Autodesk Inventor part; units mm, degrees
(part 4 of 4)
  line L785 (-17.051083, 24.790146) -> (-16.754475, 24.905018)
  line L786 (-16.754475, 24.905018) -> (-16.713136, 24.929783)
  line L787 (-16.713136, 24.929783) -> (-16.476535, 25.079515)
  line L788 (-16.476535, 25.079515) -> (-16.131349, 24.532971)
  line L789 (-16.131349, 24.532971) -> (-18.059781, 23.317391)
  line L790 (-18.059781, 23.317391) -> (-18.405157, 23.864126)
  line L791 (-18.405157, 23.864126) -> (-18.185892, 24.001666)
  line L792 (-18.185892, 24.001666) -> (-18.145696, 24.027575)
  line L793 (-18.145696, 24.027575) -> (-17.914239, 24.245697)
  line L794 (-17.914239, 24.245697) -> (-17.908905, 24.263032)
  line L795 (-17.908905, 24.263032) -> (-17.904904, 24.280749)
  line L796 (-17.904904, 24.280749) -> (-18.003012, 24.56707)
  line L797 (-18.003012, 24.56707) -> (-18.027777, 24.606313)
  line L798 (-18.027777, 24.606313) -> (-19.514058, 26.962608)
  line L799 (-10.748772, 31.507176) -> (-10.761154, 31.552705)
  line L800 (-10.761154, 31.552705) -> (-10.903649, 31.819405)
  line L801 (-10.903649, 31.819405) -> (-10.920222, 31.826454)
  line L802 (-10.920222, 31.826454) -> (-10.936796, 31.835788)
  line L803 (-10.936796, 31.835788) -> (-11.253025, 31.814071)
  line L804 (-11.253025, 31.814071) -> (-11.299507, 31.800546)
  line L805 (-11.299507, 31.800546) -> (-11.549634, 31.73368)
  line L806 (-11.549634, 31.73368) -> (-11.717083, 32.357758)
  line L807 (-11.717083, 32.357758) -> (-9.440418, 32.971549)
  line L808 (-9.440418, 32.971549) -> (-6.717982, 30.143958)
  line L809 (-6.717982, 30.143958) -> (-7.334059, 32.428053)
  line L810 (-7.334059, 32.428053) -> (-7.346442, 32.473392)
  line L811 (-7.346442, 32.473392) -> (-7.488936, 32.740092)
  line L812 (-7.488936, 32.740092) -> (-7.50551, 32.748283)
  line L813 (-7.50551, 32.748283) -> (-7.522083, 32.756665)
  line L814 (-7.522083, 32.756665) -> (-7.838313, 32.734948)
  line L815 (-7.838313, 32.734948) -> (-7.884795, 32.721613)
  line L816 (-7.884795, 32.721613) -> (-8.155495, 32.649033)
  line L817 (-8.155495, 32.649033) -> (-8.324088, 33.273492)
  line L818 (-8.324088, 33.273492) -> (-6.150483, 33.85947)
  line L819 (-6.150483, 33.85947) -> (-5.98189, 33.235201)
  line L820 (-5.98189, 33.235201) -> (-6.203061, 33.175384)
  line L821 (-6.203061, 33.175384) -> (-6.250686, 33.162811)
  line L822 (-6.250686, 33.162811) -> (-6.536055, 33.023365)
  line L823 (-6.536055, 33.023365) -> (-6.545199, 33.007744)
  line L824 (-6.545199, 33.007744) -> (-6.555486, 32.992314)
  line L825 (-6.555486, 32.992314) -> (-6.545199, 32.689609)
  line L826 (-6.545199, 32.689609) -> (-6.532816, 32.64408)
  line L827 (-6.532816, 32.64408) -> (-5.527358, 28.91809)
  line L828 (-5.527358, 28.91809) -> (-6.990779, 28.523375)
  line L829 (-6.990779, 28.523375) -> (-9.897046, 31.540132)
  line L830 (-9.897046, 31.540132) -> (-9.221343, 29.032771)
  line L831 (-9.221343, 29.032771) -> (-9.209913, 28.988575)
  line L832 (-9.209913, 28.988575) -> (-9.066276, 28.721876)
  line L833 (-9.066276, 28.721876) -> (-9.049512, 28.713303)
  line L834 (-9.049512, 28.713303) -> (-9.034272, 28.705111)
  line L835 (-9.034272, 28.705111) -> (-8.717661, 28.726828)
  line L836 (-8.717661, 28.726828) -> (-8.670417, 28.739401)
  line L837 (-8.670417, 28.739401) -> (-8.399526, 28.812553)
  line L838 (-8.399526, 28.812553) -> (-8.230933, 28.188475)
  line L839 (-8.230933, 28.188475) -> (-10.432542, 27.595258)
  line L840 (-10.432542, 27.595258) -> (-10.600753, 28.218384)
  line L841 (-10.600753, 28.218384) -> (-10.35177, 28.286583)
  line L842 (-10.35177, 28.286583) -> (-10.305288, 28.300108)
  line L843 (-10.305288, 28.300108) -> (-10.020109, 28.439554)
  line L844 (-10.020109, 28.439554) -> (-10.009632, 28.454033)
  line L845 (-10.009632, 28.454033) -> (-10.000488, 28.469653)
  line L846 (-10.000488, 28.469653) -> (-10.010775, 28.772358)
  line L847 (-10.010775, 28.772358) -> (-10.022205, 28.816744)
  line L848 (-10.022205, 28.816744) -> (-10.748772, 31.507176)
  line L849 (11.182922, -32.486917) -> (10.920222, -31.895739)
  line L850 (10.920222, -31.895739) -> (11.170349, -31.785135)
  line L851 (11.170349, -31.785135) -> (11.213783, -31.765513)
  line L852 (11.213783, -31.765513) -> (11.470196, -31.586691)
  line L853 (11.470196, -31.586691) -> (11.478387, -31.571203)
  line L854 (11.478387, -31.571203) -> (11.485626, -31.554649)
  line L855 (11.485626, -31.554649) -> (11.425809, -31.255964)
  line L856 (11.425809, -31.255964) -> (11.406949, -31.213616)
  line L857 (11.406949, -31.213616) -> (10.280332, -28.664897)
  line L858 (10.280332, -28.664897) -> (10.260901, -28.620491)
  line L859 (10.260901, -28.620491) -> (10.078974, -28.376556)
  line L860 (10.078974, -28.376556) -> (10.062401, -28.371394)
  line L861 (10.062401, -28.371394) -> (10.044875, -28.366212)
  line L862 (10.044875, -28.366212) -> (9.740075, -28.436526)
  line L863 (9.740075, -28.436526) -> (9.69645, -28.456147)
  line L864 (9.69645, -28.456147) -> (9.447467, -28.566713)
  line L865 (9.447467, -28.566713) -> (9.1861, -27.975554)
  line L866 (9.1861, -27.975554) -> (11.655171, -26.883112)
  line L867 (11.655171, -26.883112) -> (11.916537, -27.474272)
  line L868 (11.916537, -27.474272) -> (11.788521, -27.531136)
  line L869 (11.788521, -27.531136) -> (11.742991, -27.550777)
  line L870 (11.742991, -27.550777) -> (11.482387, -27.732666)
  line L871 (11.482387, -27.732666) -> (11.475339, -27.749202)
  line L872 (11.475339, -27.749202) -> (11.466957, -27.765737)
  line L873 (11.466957, -27.765737) -> (11.52506, -28.062365)
  line L874 (11.52506, -28.062365) -> (11.54449, -28.105779)
  line L875 (11.54449, -28.105779) -> (11.934063, -28.986347)
  line L876 (11.934063, -28.986347) -> (13.391388, -28.340399)
  line L877 (13.391388, -28.340399) -> (13.001815, -27.460861)
  line L878 (13.001815, -27.460861) -> (12.982004, -27.417446)
  line L879 (12.982004, -27.417446) -> (12.80141, -27.175587)
  line L880 (12.80141, -27.175587) -> (12.783693, -27.170424)
  line L881 (12.783693, -27.170424) -> (12.766167, -27.164233)
  line L882 (12.766167, -27.164233) -> (12.456033, -27.234509)
  line L883 (12.456033, -27.234509) -> (12.411646, -27.255178)
  line L884 (12.411646, -27.255178) -> (12.284583, -27.311013)
  line L885 (12.284583, -27.311013) -> (12.022836, -26.719816)
  line L886 (12.022836, -26.719816) -> (14.492097, -25.627374)
  line L887 (14.492097, -25.627374) -> (14.753653, -26.218534)
  line L888 (14.753653, -26.218534) -> (14.504479, -26.329138)
  line L889 (14.504479, -26.329138) -> (14.460093, -26.34876)
  line L890 (14.460093, -26.34876) -> (14.199679, -26.530668)
  line L891 (14.199679, -26.530668) -> (14.19244, -26.548232)
  line L892 (14.19244, -26.548232) -> (14.184059, -26.564768)
  line L893 (14.184059, -26.564768) -> (14.239875, -26.861395)
  line L894 (14.239875, -26.861395) -> (14.259687, -26.90481)
  line L895 (14.259687, -26.90481) -> (15.387066, -29.452462)
  line L896 (15.387066, -29.452462) -> (15.405926, -29.494848)
  line L897 (15.405926, -29.494848) -> (15.588805, -29.73564)
  line L898 (15.588805, -29.73564) -> (15.606141, -29.74187)
  line L899 (15.606141, -29.74187) -> (15.623857, -29.747032)
  line L900 (15.623857, -29.747032) -> (15.932849, -29.677785)
  line L901 (15.932849, -29.677785) -> (15.977426, -29.659174)
  line L902 (15.977426, -29.659174) -> (16.226409, -29.548588)
  line L903 (16.226409, -29.548588) -> (16.487775, -30.138738)
  line L904 (16.487775, -30.138738) -> (14.018704, -31.23118)
  line L905 (14.018704, -31.23118) -> (13.757339, -30.64103)
  line L906 (13.757339, -30.64103) -> (13.885355, -30.584165)
  line L907 (13.885355, -30.584165) -> (13.929741, -30.564544)
  line L908 (13.929741, -30.564544) -> (14.189392, -30.382635)
  line L909 (14.189392, -30.382635) -> (14.197584, -30.3661)
  line L910 (14.197584, -30.3661) -> (14.205014, -30.348536)
  line L911 (14.205014, -30.348536) -> (14.148054, -30.05088)
  line L912 (14.148054, -30.05088) -> (14.129194, -30.008513)
  line L913 (14.129194, -30.008513) -> (13.662279, -28.952247)
  line L914 (13.662279, -28.952247) -> (12.204002, -29.596137)
  line L915 (12.204002, -29.596137) -> (12.67225, -30.65446)
  line L916 (12.67225, -30.65446) -> (12.690729, -30.696827)
  line L917 (12.690729, -30.696827) -> (12.871514, -30.937657)
  line L918 (12.871514, -30.937657) -> (12.88923, -30.943848)
  line L919 (12.88923, -30.943848) -> (12.905613, -30.94903)
  line L920 (12.905613, -30.94903) -> (13.215747, -30.879764)
  line L921 (13.215747, -30.879764) -> (13.261276, -30.860124)
  line L922 (13.261276, -30.860124) -> (13.389293, -30.803298)
  line L923 (13.389293, -30.803298) -> (13.651992, -31.394457)
  line L924 (13.651992, -31.394457) -> (11.182922, -32.486917)
  line L925 (-31.425471, -0.940499) -> (-31.425471, 0.977646)
  line L926 (-31.425471, 0.977646) -> (-31.181573, 3.914013)
  line L927 (-31.181573, 3.914013) -> (-30.626552, 7.07155)
  line L928 (-30.626552, 7.07155) -> (-30.470494, 7.686484)
  line L929 (-30.470494, 7.686484) -> (-31.173287, 7.953184)
  line L930 (-31.173287, 7.953184) -> (-31.336583, 7.317295)
  line L931 (-31.336583, 7.317295) -> (-31.916389, 4.051554)
  line L932 (-31.916389, 4.051554) -> (-32.17063, 1.012888)
  line L933 (-32.17063, 1.012888) -> (-32.17063, -0.963359)
  line L934 (-32.17063, -0.963359) -> (-31.94224, -3.850005)
  line L935 (-31.94224, -3.850005) -> (-31.272499, -7.565517)
  line L936 (-31.272499, -7.565517) -> (-30.188344, -11.120628)
  line L937 (-30.188344, -11.120628) -> (-28.715551, -14.490001)
  line L938 (-28.715551, -14.490001) -> (-26.883112, -17.647539)
  line L939 (-26.883112, -17.647539) -> (-24.714784, -20.565161)
  line L940 (-24.714784, -20.565161) -> (-22.239465, -23.217188)
  line L941 (-22.239465, -23.217188) -> (-20.201363, -25.028976)
  line L942 (-20.201363, -25.028976) -> (-19.480987, -25.578797)
  line L943 (-19.480987, -25.578797) -> (-19.035522, -24.981427)
  line L944 (-19.035522, -24.981427) -> (-19.739362, -24.443988)
  line L945 (-19.739362, -24.443988) -> (-21.728906, -22.674586)
  line L946 (-21.728906, -22.674586) -> (-24.146332, -20.08352)
  line L947 (-24.146332, -20.08352) -> (-26.262997, -17.234154)
  line L948 (-26.262997, -17.234154) -> (-28.05202, -14.151102)
  line L949 (-28.05202, -14.151102) -> (-29.489667, -10.861358)
  line L950 (-29.489667, -10.861358) -> (-30.547989, -7.388733)
  line L951 (-30.547989, -7.388733) -> (-31.202243, -3.759899)
  line L952 (-31.202243, -3.759899) -> (-31.425471, -0.940499)
  line L953 (32.170688, -0.963359) -> (32.170688, 1.012888)
  line L954 (32.170688, 1.012888) -> (31.915418, 4.051554)
  line L955 (31.915418, 4.051554) -> (31.335726, 7.317295)
  line L956 (31.335726, 7.317295) -> (31.17323, 7.953184)
  line L957 (31.17323, 7.953184) -> (30.470475, 7.686484)
  line L958 (30.470475, 7.686484) -> (30.625542, 7.07155)
  line L959 (30.625542, 7.07155) -> (31.180659, 3.914013)
  line L960 (31.180659, 3.914013) -> (31.425451, 0.977646)
  line L961 (31.425451, 0.977646) -> (31.425451, -0.940499)
  line L962 (31.425451, -0.940499) -> (31.201233, -3.759899)
  line L963 (31.201233, -3.759899) -> (30.546865, -7.388733)
  line L964 (30.546865, -7.388733) -> (29.488638, -10.861358)
  line L965 (29.488638, -10.861358) -> (28.051887, -14.151102)
  line L966 (28.051887, -14.151102) -> (26.261949, -17.234154)
  line L967 (26.261949, -17.234154) -> (24.145304, -20.08352)
  line L968 (24.145304, -20.08352) -> (21.727859, -22.674586)
  line L969 (21.727859, -22.674586) -> (19.738467, -24.443988)
  line L970 (19.738467, -24.443988) -> (19.035522, -24.981427)
  line L971 (19.035522, -24.981427) -> (19.482054, -25.578797)
  line L972 (19.482054, -25.578797) -> (20.201382, -25.028976)
  line L973 (20.201382, -25.028976) -> (22.238399, -23.217188)
  line L974 (22.238399, -23.217188) -> (24.714708, -20.565161)
  line L975 (24.714708, -20.565161) -> (26.882217, -17.647539)
  line L976 (26.882217, -17.647539) -> (28.715589, -14.491144)
  line L977 (28.715589, -14.491144) -> (30.187392, -11.121771)
  line L978 (30.187392, -11.121771) -> (31.271337, -7.565517)
  line L979 (31.271337, -7.565517) -> (31.941326, -3.850005)
  line L980 (31.941326, -3.850005) -> (32.170688, -0.963359)
  line L981 (0.70485, 27.596211) -> (-0.705993, 27.596211)
  line L982 (-0.705993, 27.596211) -> (-2.822638, 27.454669)
  line L983 (-2.822638, 27.454669) -> (-5.562409, 27.036141)
  line L984 (-5.562409, 27.036141) -> (-8.207311, 26.355866)
  line L985 (-8.207311, 26.355866) -> (-10.742676, 25.427749)
  line L986 (-10.742676, 25.427749) -> (-13.154787, 24.266271)
  line L987 (-13.154787, 24.266271) -> (-15.4305, 22.883241)
  line L988 (-15.4305, 22.883241) -> (-17.554575, 21.294661)
  line L989 (-17.554575, 21.294661) -> (-19.515087, 19.514058)
  line L990 (-19.515087, 19.514058) -> (-21.295862, 17.553432)
  line L991 (-21.295862, 17.553432) -> (-22.884403, 15.429357)
  line L992 (-22.884403, 15.429357) -> (-24.267243, 13.153834)
  line L993 (-24.267243, 13.153834) -> (-25.42895, 10.741533)
  line L994 (-25.42895, 10.741533) -> (-26.357047, 8.206359)
  line L995 (-26.357047, 8.206359) -> (-27.037113, 5.561457)
  line L996 (-27.037113, 5.561457) -> (-27.455679, 2.821495)
  line L997 (-27.455679, 2.821495) -> (-27.597278, 0.70485)
  line L998 (-27.597278, 0.70485) -> (-27.597278, -0.705993)
  line L999 (-27.597278, -0.705993) -> (-27.455679, -2.821496)
  line L1000 (-27.455679, -2.821496) -> (-27.037113, -5.56241)
  line L1001 (-27.037113, -5.56241) -> (-26.357047, -8.206359)
  line L1002 (-26.357047, -8.206359) -> (-25.42895, -10.742676)
  line L1003 (-25.42895, -10.742676) -> (-24.267243, -13.154787)
  line L1004 (-24.267243, -13.154787) -> (-22.884403, -15.429547)
  line L1005 (-22.884403, -15.429547) -> (-21.295862, -17.554575)
  line L1006 (-21.295862, -17.554575) -> (-19.515087, -19.514058)
  line L1007 (-19.515087, -19.514058) -> (-17.554575, -21.294833)
  line L1008 (-17.554575, -21.294833) -> (-15.4305, -22.883355)
  line L1009 (-15.4305, -22.883355) -> (-13.154787, -24.266214)
  line L1010 (-13.154787, -24.266214) -> (-10.742676, -25.427921)
  line L1011 (-10.742676, -25.427921) -> (-8.207311, -26.356018)
  line L1012 (-8.207311, -26.356018) -> (-5.562409, -27.036084)
  line L1013 (-5.562409, -27.036084) -> (-2.822638, -27.45465)
  line L1014 (-2.822638, -27.45465) -> (-0.705993, -27.597278)
  line L1015 (-0.705993, -27.597278) -> (0.70485, -27.597278)
  line L1016 (0.70485, -27.597278) -> (2.821496, -27.45465)
  line L1017 (2.821496, -27.45465) -> (5.561457, -27.036084)
  line L1018 (5.561457, -27.036084) -> (8.206359, -26.356018)
  line L1019 (8.206359, -26.356018) -> (10.741533, -25.427921)
  line L1020 (10.741533, -25.427921) -> (13.153835, -24.266214)
  line L1021 (13.153835, -24.266214) -> (15.429357, -22.883355)
  line L1022 (15.429357, -22.883355) -> (17.553432, -21.294833)
  line L1023 (17.553432, -21.294833) -> (19.514058, -19.514058)
  line L1024 (19.514058, -19.514058) -> (21.294662, -17.554575)
  line L1025 (21.294662, -17.554575) -> (22.883241, -15.429547)
  line L1026 (22.883241, -15.429547) -> (24.266271, -13.154787)
  line L1027 (24.266271, -13.154787) -> (25.42775, -10.742676)
  line L1028 (25.42775, -10.742676) -> (26.355866, -8.206359)
  line L1029 (26.355866, -8.206359) -> (27.036141, -5.56241)
  line L1030 (27.036141, -5.56241) -> (27.454669, -2.821496)
  line L1031 (27.454669, -2.821496) -> (27.597354, -0.705993)
  line L1032 (27.597354, -0.705993) -> (27.597354, 0.70485)
  line L1033 (27.597354, 0.70485) -> (27.454669, 2.821495)
  line L1034 (27.454669, 2.821495) -> (27.036141, 5.561457)
  line L1035 (27.036141, 5.561457) -> (26.355866, 8.206359)
  line L1036 (26.355866, 8.206359) -> (25.42775, 10.741533)
  line L1037 (25.42775, 10.741533) -> (24.266271, 13.153834)
  line L1038 (24.266271, 13.153834) -> (22.883241, 15.429357)
  line L1039 (22.883241, 15.429357) -> (21.294662, 17.553432)
  line L1040 (21.294662, 17.553432) -> (19.514058, 19.514058)
  line L1041 (19.514058, 19.514058) -> (17.553432, 21.294661)
  line L1042 (17.553432, 21.294661) -> (15.429357, 22.883241)
  line L1043 (15.429357, 22.883241) -> (13.153835, 24.266271)
  line L1044 (13.153835, 24.266271) -> (10.741533, 25.427749)
  line L1045 (10.741533, 25.427749) -> (8.206359, 26.355866)
  line L1046 (8.206359, 26.355866) -> (5.561457, 27.036141)
  line L1047 (5.561457, 27.036141) -> (2.821496, 27.454669)
  line L1048 (2.821496, 27.454669) -> (0.70485, 27.596211)
  line L1049 (1.267016, -25.161259) -> (-1.268158, -25.161259)
  line L1050 (-1.268158, -25.161259) -> (-5.071491, -24.649671)
  line L1051 (-5.071491, -24.649671) -> (-9.794938, -23.183088)
  line L1052 (-9.794938, -23.183088) -> (-14.068425, -20.863846)
  line L1053 (-14.068425, -20.863846) -> (-17.792128, -17.791176)
  line L1054 (-17.792128, -17.791176) -> (-20.864874, -14.068425)
  line L1055 (-20.864874, -14.068425) -> (-23.184117, -9.793796)
  line L1056 (-23.184117, -9.793796) -> (-24.6507, -5.071491)
  line L1057 (-24.6507, -5.071491) -> (-25.161259, -1.268159)
  line L1058 (-25.161259, -1.268159) -> (-25.161259, 1.267015)
  line L1059 (-25.161259, 1.267015) -> (-24.6507, 5.070538)
  line L1060 (-24.6507, 5.070538) -> (-23.184117, 9.793795)
  line L1061 (-23.184117, 9.793795) -> (-20.864874, 14.067282)
  line L1062 (-20.864874, 14.067282) -> (-17.792128, 17.791176)
  line L1063 (-17.792128, 17.791176) -> (-14.068425, 20.86375)
  line L1064 (-14.068425, 20.86375) -> (-9.794938, 23.183088)
  line L1065 (-9.794938, 23.183088) -> (-5.071491, 24.649557)
  line L1066 (-5.071491, 24.649557) -> (-1.268158, 25.160287)
  line L1067 (-1.268158, 25.160287) -> (1.267016, 25.160287)
  line L1068 (1.267016, 25.160287) -> (5.070539, 24.649557)
  line L1069 (5.070539, 24.649557) -> (9.793795, 23.183088)
  line L1070 (9.793795, 23.183088) -> (14.067282, 20.86375)
  line L1071 (14.067282, 20.86375) -> (17.791176, 17.791176)
  line L1072 (17.791176, 17.791176) -> (20.86375, 14.067282)
  line L1073 (20.86375, 14.067282) -> (23.183088, 9.793795)
  line L1074 (23.183088, 9.793795) -> (24.649557, 5.070538)
  line L1075 (24.649557, 5.070538) -> (25.161431, 1.267015)
  line L1076 (25.161431, 1.267015) -> (25.161431, -1.268159)
  line L1077 (25.161431, -1.268159) -> (24.649557, -5.071491)
  line L1078 (24.649557, -5.071491) -> (23.183088, -9.793796)
  line L1079 (23.183088, -9.793796) -> (20.86375, -14.068425)
  line L1080 (20.86375, -14.068425) -> (17.791176, -17.791176)
  line L1081 (17.791176, -17.791176) -> (14.067282, -20.863846)
  line L1082 (14.067282, -20.863846) -> (9.793795, -23.183088)
  line L1083 (9.793795, -23.183088) -> (5.070539, -24.649671)
  line L1084 (5.070539, -24.649671) -> (1.267016, -25.161259)
  line L1085 (-20.470063, -8.89235) -> (-20.470063, -8.548497)
  line L1086 (-18.67281, -8.89235) -> (-20.470063, -8.89235)
  line L1087 (-18.67281, -8.548497) -> (-18.67281, -8.89235)
  line L1088 (-18.67281, -8.548497) -> (-18.985992, -8.548497)
  line L1089 (-19.189522, -8.507921) -> (-18.985992, -8.548497)
  line L1090 (-19.19779, -8.500872) -> (-19.189522, -8.507921)
  line L1091 (-19.207086, -8.492681) -> (-19.19779, -8.500872)
  line L1092 (-19.25153, -8.331136) -> (-19.207086, -8.492681)
  line L1093 (-19.25153, -8.331136) -> (-19.25153, -5.953125)
  line L1094 (-19.639121, -5.953125) -> (-19.25153, -5.953125)
  line L1095 (-19.656685, -5.990463) -> (-19.639121, -5.953125)
  line L1096 (-19.901611, -6.262116) -> (-19.656685, -5.990463)
  line L1097 (-19.933653, -6.279642) -> (-19.901611, -6.262116)
  line L1098 (-19.965695, -6.296216) -> (-19.933653, -6.279642)
  line L1099 (-20.413218, -6.394514) -> (-19.965695, -6.296216)
  line L1100 (-20.470063, -6.397562) -> (-20.413218, -6.394514)
  line L1101 (-20.470063, -6.736461) -> (-20.470063, -6.397562)
  line L1102 (-19.88199, -6.736461) -> (-20.470063, -6.736461)
  line L1103 (-19.88199, -6.736461) -> (-19.88199, -8.32085)
  line L1104 (-19.936777, -8.486203) -> (-19.88199, -8.32085)
  line L1105 (-19.947103, -8.495538) -> (-19.936777, -8.486203)
  line L1106 (-19.958475, -8.50392) -> (-19.947103, -8.495538)
  line L1107 (-20.179646, -8.548497) -> (-19.958475, -8.50392)
  line L1108 (-20.179646, -8.548497) -> (-20.470063, -8.548497)
  line L1109 (14.425803, -8.89235) -> (14.425803, -8.548497)
  line L1110 (16.223171, -8.89235) -> (14.425803, -8.89235)
  line L1111 (16.223171, -8.548497) -> (16.223171, -8.89235)
  line L1112 (16.223171, -8.548497) -> (15.911322, -8.548497)
  line L1113 (15.706535, -8.507921) -> (15.911322, -8.548497)
  line L1114 (15.698343, -8.500872) -> (15.706535, -8.507921)
  line L1115 (15.689009, -8.492681) -> (15.698343, -8.500872)
  line L1116 (15.645575, -8.331136) -> (15.689009, -8.492681)
  line L1117 (15.645575, -8.331136) -> (15.645575, -5.953125)
  line L1118 (15.256954, -5.953125) -> (15.645575, -5.953125)
  line L1119 (15.239428, -5.990463) -> (15.256954, -5.953125)
  line L1120 (14.994445, -6.262116) -> (15.239428, -5.990463)
  line L1121 (14.963585, -6.279642) -> (14.994445, -6.262116)
  line L1122 (14.93158, -6.296216) -> (14.963585, -6.279642)
  line L1123 (14.482763, -6.394514) -> (14.93158, -6.296216)
  line L1124 (14.425803, -6.397562) -> (14.482763, -6.394514)
  line L1125 (14.425803, -6.736461) -> (14.425803, -6.397562)
  line L1126 (15.014067, -6.736461) -> (14.425803, -6.736461)
  line L1127 (15.014067, -6.736461) -> (15.014067, -8.32085)
  line L1128 (14.960346, -8.486203) -> (15.014067, -8.32085)
  line L1129 (14.950059, -8.495538) -> (14.960346, -8.486203)
  line L1130 (14.938629, -8.50392) -> (14.950059, -8.495538)
  line L1131 (14.717458, -8.548497) -> (14.938629, -8.50392)
  line L1132 (14.717458, -8.548497) -> (14.425803, -8.548497)
  line L1133 (17.692878, -8.441817) -> (17.713643, -8.458391)
  line L1134 (17.761268, -8.441817) -> (17.692878, -8.441817)
  line L1135 (17.966817, -8.361426) -> (17.761268, -8.441817)
  line L1136 (17.985677, -8.345805) -> (17.966817, -8.361426)
  line L1137 (18.003012, -8.329041) -> (17.985677, -8.345805)
  line L1138 (18.094071, -8.150542) -> (18.003012, -8.329041)
  line L1139 (18.094071, -8.150542) -> (18.094071, -8.026337)
  line L1140 (18.00206, -7.851839) -> (18.094071, -8.026337)
  line L1141 (17.983391, -7.836217) -> (18.00206, -7.851839)
  line L1142 (17.964722, -7.819835) -> (17.983391, -7.836217)
  line L1143 (17.769459, -7.740205) -> (17.964722, -7.819835)
  line L1144 (17.769459, -7.740205) -> (17.625822, -7.740205)
  line L1145 (17.410938, -7.843647) -> (17.625822, -7.740205)
  line L1146 (17.391126, -7.864221) -> (17.410938, -7.843647)
  line L1147 (17.370361, -7.884795) -> (17.391126, -7.864221)
  line L1148 (17.267301, -8.093583) -> (17.370361, -7.884795)
  line L1149 (17.267301, -8.093583) -> (17.267301, -8.30561)
  line L1150 (17.545241, -8.710613) -> (17.267301, -8.30561)
  line L1151 (17.600866, -8.748712) -> (17.545241, -8.710613)
  line L1152 (17.655731, -8.786051) -> (17.600866, -8.748712)
  line L1153 (18.253139, -8.974074) -> (17.655731, -8.786051)
  line L1154 (18.253139, -8.974074) -> (18.601563, -8.974074)
  line L1155 (18.992088, -8.897684) -> (18.601563, -8.974074)
  line L1156 (19.333083, -8.722042) -> (18.992088, -8.897684)
  line L1157 (19.3889, -8.672322) -> (19.333083, -8.722042)
  line L1158 (19.444716, -8.621649) -> (19.3889, -8.672322)
  line L1159 (19.639979, -8.315896) -> (19.444716, -8.621649)
  line L1160 (19.723799, -7.967472) -> (19.639979, -8.315896)
  line L1161 (19.723799, -7.967472) -> (19.723799, -7.678293)
  line L1162 (19.447955, -7.160133) -> (19.723799, -7.678293)
  line L1163 (19.393091, -7.111746) -> (19.447955, -7.160133)
  line L1164 (19.337274, -7.062026) -> (19.393091, -7.111746)
  line L1165 (18.758345, -6.818376) -> (19.337274, -7.062026)
  line L1166 (18.758345, -6.818376) -> (18.462879, -6.818376)
  line L1167 (18.2118, -6.853238) -> (18.462879, -6.818376)
  line L1168 (18.181892, -6.860667) -> (18.2118, -6.853238)
  line L1169 (18.15103, -6.867716) -> (18.181892, -6.860667)
  line L1170 (17.842992, -6.975158) -> (18.15103, -6.867716)
  line L1171 (17.81175, -6.989826) -> (17.842992, -6.975158)
  line L1172 (17.849088, -6.551676) -> (17.81175, -6.989826)
  line L1173 (17.879949, -6.555486) -> (17.849088, -6.551676)
  line L1174 (18.138458, -6.585776) -> (17.879949, -6.555486)
  line L1175 (18.159222, -6.587681) -> (18.138458, -6.585776)
  line L1176 (18.178653, -6.588633) -> (18.159222, -6.587681)
  line L1177 (18.320195, -6.597968) -> (18.178653, -6.588633)
  line L1178 (18.320195, -6.597968) -> (18.564225, -6.597968)
  line L1179 (19.13363, -6.457378) -> (18.564225, -6.597968)
  line L1180 (19.18335, -6.429566) -> (19.13363, -6.457378)
  line L1181 (19.23288, -6.401562) -> (19.18335, -6.429566)
  line L1182 (19.559588, -5.972747) -> (19.23288, -6.401562)
  line L1183 (19.575971, -5.914835) -> (19.559588, -5.972747)
  line L1184 (19.536918, -5.927217) -> (19.575971, -5.914835)
  line L1185 (19.124295, -6.019229) -> (19.536918, -5.927217)
  line L1186 (19.082004, -6.025325) -> (19.124295, -6.019229)
  line L1187 (19.03857, -6.031611) -> (19.082004, -6.025325)
  line L1188 (18.677953, -6.062663) -> (19.03857, -6.031611)
  line L1189 (18.677953, -6.062663) -> (18.423636, -6.062663)
  line L1190 (18.066068, -6.030659) -> (18.423636, -6.062663)
  line L1191 (18.025872, -6.024563) -> (18.066068, -6.030659)
  line L1192 (17.984534, -6.018276) -> (18.025872, -6.024563)
  line L1193 (17.583341, -5.922264) -> (17.984534, -6.018276)
  line L1194 (17.544288, -5.909691) -> (17.583341, -5.922264)
  line L1195 (17.39627, -7.457885) -> (17.544288, -5.909691)
  line L1196 (17.721072, -7.472363) -> (17.39627, -7.457885)
  line L1197 (17.742789, -7.445692) -> (17.721072, -7.472363)
  line L1198 (17.975199, -7.254431) -> (17.742789, -7.445692)
  line L1199 (17.999964, -7.241858) -> (17.975199, -7.254431)
  line L1200 (18.024729, -7.228332) -> (17.999964, -7.241858)
  line L1201 (18.244947, -7.16642) -> (18.024729, -7.228332)
  line L1202 (18.244947, -7.16642) -> (18.447639, -7.16642)
  line L1203 (18.807113, -7.330821) -> (18.447639, -7.16642)
  line L1204 (18.838164, -7.363968) -> (18.807113, -7.330821)
  line L1205 (18.868263, -7.395972) -> (18.838164, -7.363968)
  line L1206 (19.021235, -7.777353) -> (18.868263, -7.395972)
  line L1207 (19.021235, -7.777353) -> (19.021235, -8.041957)
  line L1208 (18.861977, -8.4201) -> (19.021235, -8.041957)
  line L1209 (18.830925, -8.452104) -> (18.861977, -8.4201)
  line L1210 (18.798921, -8.484108) -> (18.830925, -8.452104)
  line L1211 (18.432018, -8.643366) -> (18.798921, -8.484108)
  line L1212 (18.432018, -8.643366) -> (18.224183, -8.643366)
  line L1213 (17.997678, -8.602218) -> (18.224183, -8.643366)
  line L1214 (17.973104, -8.593646) -> (17.997678, -8.602218)
  line L1215 (17.947196, -8.584311) -> (17.973104, -8.593646)
  line L1216 (17.713643, -8.458391) -> (17.947196, -8.584311)
  line L1217 (-16.940593, -8.581454) -> (-16.926115, -8.590788)
  line L1218 (-16.923068, -8.574024) -> (-16.940593, -8.581454)
  line L1219 (-16.787622, -8.485251) -> (-16.923068, -8.574024)
  line L1220 (-16.778287, -8.474774) -> (-16.787622, -8.485251)
  line L1221 (-16.770096, -8.463534) -> (-16.778287, -8.474774)
  line L1222 (-16.725519, -8.349996) -> (-16.770096, -8.463534)
  line L1223 (-16.725519, -8.349996) -> (-16.725519, -8.255889)
  line L1224 (-16.807244, -8.100822) -> (-16.725519, -8.255889)
  line L1225 (-16.822674, -8.086154) -> (-16.807244, -8.100822)
  line L1226 (-16.839247, -8.071866) -> (-16.822674, -8.086154)
  line L1227 (-17.011841, -7.998333) -> (-16.839247, -8.071866)
  line L1228 (-17.011841, -7.998333) -> (-17.142142, -7.998333)
  line L1229 (-17.345787, -8.083296) -> (-17.142142, -7.998333)
  line L1230 (-17.364265, -8.100822) -> (-17.345787, -8.083296)
  line L1231 (-17.382934, -8.117396) -> (-17.364265, -8.100822)
  line L1232 (-17.477041, -8.300276) -> (-17.382934, -8.117396)
  line L1233 (-17.477041, -8.300276) -> (-17.477041, -8.468868)
  line L1234 (-17.257966, -8.775764) -> (-17.477041, -8.468868)
  line L1235 (-17.213389, -8.805672) -> (-17.257966, -8.775764)
  line L1236 (-17.169956, -8.834628) -> (-17.213389, -8.805672)
  line L1237 (-16.713136, -8.983409) -> (-17.169956, -8.834628)
  line L1238 (-16.713136, -8.983409) -> (-16.399954, -8.983409)
  line L1239 (-15.961805, -8.87711) -> (-16.399954, -8.983409)
  line L1240 (-15.580423, -8.628888) -> (-15.961805, -8.87711)
  line L1241 (-15.517368, -8.558784) -> (-15.580423, -8.628888)
  line L1242 (-15.455455, -8.487347) -> (-15.517368, -8.558784)
  line L1243 (-15.238285, -8.053197) -> (-15.455455, -8.487347)
  line L1244 (-15.144369, -7.556945) -> (-15.238285, -8.053197)
  line L1245 (-15.144369, -7.556945) -> (-15.144369, -7.233666)
  line L1246 (-15.229141, -6.761416) -> (-15.144369, -7.233666)
  line L1247 (-15.424404, -6.356033) -> (-15.229141, -6.761416)
  line L1248 (-15.480221, -6.291072) -> (-15.424404, -6.356033)
  line L1249 (-15.536989, -6.225921) -> (-15.480221, -6.291072)
  line L1250 (-15.886366, -5.997512) -> (-15.536989, -6.225921)
  line L1251 (-16.294608, -5.900547) -> (-15.886366, -5.997512)
  line L1252 (-16.294608, -5.900547) -> (-16.638841, -5.900547)
  line L1253 (-17.265015, -6.132957) -> (-16.638841, -5.900547)
  line L1254 (-17.319879, -6.179439) -> (-17.265015, -6.132957)
  line L1255 (-17.375695, -6.225921) -> (-17.319879, -6.179439)
  line L1256 (-17.653635, -6.736461) -> (-17.375695, -6.225921)
  line L1257 (-17.653635, -6.736461) -> (-17.653635, -7.076504)
  line L1258 (-17.410747, -7.538466) -> (-17.653635, -7.076504)
  line L1259 (-17.36217, -7.583043) -> (-17.410747, -7.538466)
  line L1260 (-17.314735, -7.627429) -> (-17.36217, -7.583043)
  line L1261 (-16.81753, -7.850695) -> (-17.314735, -7.627429)
  line L1262 (-16.81753, -7.850695) -> (-16.544734, -7.850695)
  line L1263 (-16.2687, -7.793736) -> (-16.544734, -7.850695)
  line L1264 (-16.237839, -7.782496) -> (-16.2687, -7.793736)
  line L1265 (-16.206787, -7.771067) -> (-16.237839, -7.782496)
  line L1266 (-15.900844, -7.601521) -> (-16.206787, -7.771067)
  line L1267 (-15.870936, -7.579043) -> (-15.900844, -7.601521)
  line L1268 (-15.871888, -7.672959) -> (-15.870936, -7.579043)
  line L1269 (-16.019716, -8.37457) -> (-15.871888, -7.672959)
  line L1270 (-16.047529, -8.4201) -> (-16.019716, -8.37457)
  line L1271 (-16.076485, -8.464486) -> (-16.047529, -8.4201)
  line L1272 (-16.441293, -8.692134) -> (-16.076485, -8.464486)
  line L1273 (-16.441293, -8.692134) -> (-16.617124, -8.692134)
  line L1274 (-16.749331, -8.668322) -> (-16.617124, -8.692134)
  line L1275 (-16.763809, -8.664131) -> (-16.749331, -8.668322)
  line L1276 (-16.77943, -8.658987) -> (-16.763809, -8.664131)
  line L1277 (-16.926115, -8.590788) -> (-16.77943, -8.658987)
  line L1278 (-15.909036, -6.753035) -> (-15.909036, -6.963918)
  line L1279 (-16.017621, -7.258621) -> (-15.909036, -6.963918)
  line L1280 (-16.039338, -7.284149) -> (-16.017621, -7.258621)
  line L1281 (-16.061055, -7.310247) -> (-16.039338, -7.284149)
  line L1282 (-16.303943, -7.439216) -> (-16.061055, -7.310247)
  line L1283 (-16.303943, -7.439216) -> (-16.487965, -7.439216)
  line L1284 (-16.773144, -7.3112) -> (-16.487965, -7.439216)
  line L1285 (-16.795813, -7.286434) -> (-16.773144, -7.3112)
  line L1286 (-16.819626, -7.260526) -> (-16.795813, -7.286434)
  line L1287 (-16.936402, -6.951345) -> (-16.819626, -7.260526)
  line L1288 (-16.936402, -6.951345) -> (-16.936402, -6.737604)
  line L1289 (-16.828008, -6.429566) -> (-16.936402, -6.737604)
  line L1290 (-16.805148, -6.404801) -> (-16.828008, -6.429566)
  line L1291 (-16.783431, -6.378893) -> (-16.805148, -6.404801)
  line L1292 (-16.520922, -6.253925) -> (-16.783431, -6.378893)
  line L1293 (-16.520922, -6.253925) -> (-16.335946, -6.253925)
  line L1294 (-16.065246, -6.385179) -> (-16.335946, -6.253925)
  line L1295 (-16.042386, -6.411849) -> (-16.065246, -6.385179)
  line L1296 (-16.020669, -6.437757) -> (-16.042386, -6.411849)
  line L1297 (-15.909036, -6.753035) -> (-16.020669, -6.437757)
  line L1298 (1.435608, -12.052935) -> (2.963037, -14.304074)
  line L1299 (2.963037, -14.304074) -> (3.054096, -14.131481)
  line L1300 (3.054096, -14.131481) -> (3.477959, -13.134022)
  line L1301 (3.477959, -13.134022) -> (3.854958, -11.942445)
  line L1302 (3.854958, -11.942445) -> (3.923157, -11.673649)
  line L1303 (3.923157, -11.673649) -> (4.728401, -9.001125)
  line L1304 (4.728401, -9.001125) -> (4.776978, -9.177528)
  line L1305 (4.776978, -9.177528) -> (5.028057, -9.683305)
  line L1306 (5.028057, -9.683305) -> (5.437442, -10.062401)
  line L1307 (5.437442, -10.062401) -> (5.922074, -10.187559)
  line L1308 (5.922074, -10.187559) -> (6.446139, -10.110026)
  line L1309 (6.446139, -10.110026) -> (6.974205, -9.877425)
  line L1310 (6.974205, -9.877425) -> (7.470267, -9.540621)
  line L1311 (7.470267, -9.540621) -> (7.900225, -9.149906)
  line L1312 (7.900225, -9.149906) -> (8.155495, -8.85825)
  line L1313 (8.155495, -8.85825) -> (8.229029, -8.754047)
  line L1314 (8.229029, -8.754047) -> (8.690039, -8.088249)
  line L1315 (8.690039, -8.088249) -> (9.885616, -5.960174)
  line L1316 (9.885616, -5.960174) -> (11.095101, -3.139821)
  line L1317 (11.095101, -3.139821) -> (11.871008, -0.474345)
  line L1318 (11.871008, -0.474345) -> (12.186475, 1.269111)
  line L1319 (12.186475, 1.269111) -> (12.228766, 1.854136)
  line L1320 (12.228766, 1.854136) -> (12.233719, 1.745742)
  line L1321 (12.233719, 1.745742) -> (12.257532, 0.599503)
  line L1322 (12.257532, 0.599503) -> (12.257532, 0.478726)
  line L1323 (12.257532, 0.478726) -> (12.255437, -0.115634)
  line L1324 (12.255437, -0.115634) -> (12.008549, -1.901571)
  line L1325 (12.008549, -1.901571) -> (11.267504, -4.741926)
  line L1326 (11.267504, -4.741926) -> (10.014014, -7.805166)
  line L1327 (10.014014, -7.805166) -> (8.731187, -10.131743)
  line L1328 (8.731187, -10.131743) -> (8.229029, -10.856024)
  line L1329 (8.229029, -10.856024) -> (8.162925, -10.950321)
  line L1330 (8.162925, -10.950321) -> (7.954137, -11.226356)
  line L1331 (7.954137, -11.226356) -> (7.590282, -11.667554)
  line L1332 (7.590282, -11.667554) -> (7.162228, -12.131611)
  line L1333 (7.162228, -12.131611) -> (6.693217, -12.57281)
  line L1334 (6.693217, -12.57281) -> (6.208395, -12.941808)
  line L1335 (6.208395, -12.941808) -> (5.731955, -13.193078)
  line L1336 (5.731955, -13.193078) -> (5.287518, -13.278802)
  line L1337 (5.287518, -13.278802) -> (4.978337, -13.207555)
  line L1338 (4.978337, -13.207555) -> (4.900041, -13.151739)
  line L1339 (4.900041, -13.151739) -> (4.910328, -13.227177)
  line L1340 (4.910328, -13.227177) -> (5.110734, -13.861732)
  line L1341 (5.110734, -13.861732) -> (5.144834, -13.927836)
  line L1342 (5.144834, -13.927836) -> (6.803707, -17.177195)
  line L1343 (6.803707, -17.177195) -> (6.803707, -14.610017)
  line L1344 (6.803707, -14.610017) -> (6.829615, -14.613065)
  line L1345 (6.829615, -14.613065) -> (7.101459, -14.645069)
  line L1346 (7.101459, -14.645069) -> (7.130224, -14.648117)
  line L1347 (7.130224, -14.648117) -> (7.284339, -14.665833)
  line L1348 (7.284339, -14.665833) -> (8.410765, -14.740128)
  line L1349 (8.410765, -14.740128) -> (10.014966, -14.79804)
  line L1350 (10.014966, -14.79804) -> (10.407586, -14.807375)
  line L1351 (10.407586, -14.807375) -> (10.407586, -19.352819)
  line L1352 (10.407586, -19.352819) -> (-10.628757, -19.352819)
  line L1353 (-10.628757, -19.352819) -> (-10.628757, -14.807375)
  line L1354 (-10.628757, -14.807375) -> (-10.244328, -14.807375)
  line L1355 (-10.244328, -14.807375) -> (-9.089707, -14.779371)
  line L1356 (-9.089707, -14.779371) -> (-7.975854, -14.712315)
  line L1357 (-7.975854, -14.712315) -> (-7.775257, -14.692694)
  line L1358 (-7.775257, -14.692694) -> (-7.705915, -14.685454)
  line L1359 (-7.705915, -14.685454) -> (-7.051738, -14.602778)
  line L1360 (-7.051738, -14.602778) -> (-6.990779, -14.593443)
  line L1361 (-6.990779, -14.593443) -> (-6.990779, -17.177195)
  line L1362 (-6.990779, -17.177195) -> (-5.38372, -14.030135)
  line L1363 (-5.38372, -14.030135) -> (-5.346383, -13.955649)
  line L1364 (-5.346383, -13.955649) -> (-5.071491, -13.174409)
  line L1365 (-5.071491, -13.174409) -> (-5.060061, -13.094779)
  line L1366 (-5.060061, -13.094779) -> (-5.134546, -13.162026)
  line L1367 (-5.134546, -13.162026) -> (-5.443537, -13.272516)
  line L1368 (-5.443537, -13.272516) -> (-5.892355, -13.217843)
  line L1369 (-5.892355, -13.217843) -> (-6.377749, -12.982194)
  line L1370 (-6.377749, -12.982194) -> (-6.874955, -12.614148)
  line L1371 (-6.874955, -12.614148) -> (-7.358634, -12.167807)
  line L1372 (-7.358634, -12.167807) -> (-7.802118, -11.691366)
  line L1373 (-7.802118, -11.691366) -> (-8.177212, -11.236642)
  line L1374 (-8.177212, -11.236642) -> (-8.392287, -10.953179)
  line L1375 (-8.392287, -10.953179) -> (-8.459533, -10.856024)
  line L1376 (-8.459533, -10.856024) -> (-8.961691, -10.131743)
  line L1377 (-8.961691, -10.131743) -> (-10.245471, -7.805166)
  line L1378 (-10.245471, -7.805166) -> (-11.498961, -4.741926)
  line L1379 (-11.498961, -4.741926) -> (-12.241149, -1.901571)
  line L1380 (-12.241149, -1.901571) -> (-12.487084, -0.115634)
  line L1381 (-12.487084, -0.115634) -> (-12.48918, 0.478726)
  line L1382 (-12.48918, 0.478726) -> (-12.490132, 0.599503)
  line L1383 (-12.490132, 0.599503) -> (-12.465367, 1.745742)
  line L1384 (-12.465367, 1.745742) -> (-12.459081, 1.854136)
  line L1385 (-12.459081, 1.854136) -> (-12.41679, 1.269111)
  line L1386 (-12.41679, 1.269111) -> (-12.102655, -0.474345)
  line L1387 (-12.102655, -0.474345) -> (-11.326558, -3.139821)
  line L1388 (-11.326558, -3.139821) -> (-10.117074, -5.960174)
  line L1389 (-10.117074, -5.960174) -> (-8.921496, -8.088249)
  line L1390 (-8.921496, -8.088249) -> (-8.459533, -8.754047)
  line L1391 (-8.459533, -8.754047) -> (-8.386953, -8.85825)
  line L1392 (-8.386953, -8.85825) -> (-8.132826, -9.149906)
  line L1393 (-8.132826, -9.149906) -> (-7.702867, -9.540621)
  line L1394 (-7.702867, -9.540621) -> (-7.205662, -9.877425)
  line L1395 (-7.205662, -9.877425) -> (-6.678549, -10.110026)
  line L1396 (-6.678549, -10.110026) -> (-6.154674, -10.187559)
  line L1397 (-6.154674, -10.187559) -> (-5.670042, -10.062401)
  line L1398 (-5.670042, -10.062401) -> (-5.259705, -9.683305)
  line L1399 (-5.259705, -9.683305) -> (-5.007483, -9.178671)
  line L1400 (-5.007483, -9.178671) -> (-4.958905, -9.001125)
  line L1401 (-4.958905, -9.001125) -> (-4.153662, -11.673649)
  line L1402 (-4.153662, -11.673649) -> (-4.082605, -11.956923)
  line L1403 (-4.082605, -11.956923) -> (-3.681412, -13.206412)
  line L1404 (-3.681412, -13.206412) -> (-3.227641, -14.241018)
  line L1405 (-3.227641, -14.241018) -> (-3.129534, -14.417802)
  line L1406 (-3.129534, -14.417802) -> (-1.523429, -12.052935)
  line L1407 (-1.523429, -12.052935) -> (-2.357437, -15.50289)
  line L1408 (-2.357437, -15.50289) -> (-2.234375, -15.635288)
  line L1409 (-2.234375, -15.635288) -> (-1.584388, -16.134398)
  line L1410 (-1.584388, -16.134398) -> (-0.900112, -16.433102)
  line L1411 (-0.900112, -16.433102) -> (-0.758571, -16.465106)
  line L1412 (-0.758571, -16.465106) -> (-0.027813, -12.36726)
  line L1413 (-0.027813, -12.36726) -> (0.783336, -16.399002)
  line L1414 (0.783336, -16.399002) -> (0.911543, -16.356711)
  line L1415 (0.911543, -16.356711) -> (1.534859, -16.02486)
  line L1416 (1.534859, -16.02486) -> (2.126933, -15.51432)
  line L1417 (2.126933, -15.51432) -> (2.240661, -15.384018)
  line L1418 (2.240661, -15.384018) -> (1.435608, -12.052935)
  line L1419 (17.172051, 16.11268) -> (17.172051, 2.422588)
  line L1420 (17.172051, 2.422588) -> (12.363259, 2.422588)
  line L1421 (12.363259, 2.422588) -> (12.363259, 2.817304)
  line L1422 (12.363259, 2.817304) -> (12.3063, 3.999738)
  line L1423 (12.3063, 3.999738) -> (12.175045, 5.195697)
  line L1424 (12.175045, 5.195697) -> (12.137708, 5.418582)
  line L1425 (12.137708, 5.418582) -> (9.773222, 1.311592)
  line L1426 (9.773222, 1.311592) -> (11.41838, 8.127682)
  line L1427 (11.41838, 8.127682) -> (11.292459, 8.4201)
  line L1428 (11.292459, 8.4201) -> (10.479786, 9.628441)
  line L1429 (10.479786, 9.628441) -> (9.415463, 10.516171)
  line L1430 (9.415463, 10.516171) -> (9.16324, 10.648378)
  line L1431 (9.16324, 10.648378) -> (7.332916, 4.981575)
  line L1432 (7.332916, 4.981575) -> (7.258621, 11.266551)
  line L1433 (7.258621, 11.266551) -> (7.070407, 11.299507)
  line L1434 (7.070407, 11.299507) -> (6.058472, 11.397805)
  line L1435 (6.058472, 11.397805) -> (4.950524, 11.415522)
  line L1436 (4.950524, 11.415522) -> (4.714875, 11.406949)
  line L1437 (4.714875, 11.406949) -> (4.725162, -4.028885)
  line L1438 (4.725162, -4.028885) -> (4.725162, -4.259199)
  line L1439 (4.725162, -4.259199) -> (4.528947, -4.953762)
  line L1440 (4.528947, -4.953762) -> (4.022408, -5.571935)
  line L1441 (4.022408, -5.571935) -> (3.332226, -5.801296)
  line L1442 (3.332226, -5.801296) -> (2.736914, -5.668899)
  line L1443 (2.736914, -5.668899) -> (2.579751, -5.564505)
  line L1444 (2.579751, -5.564505) -> (2.432876, -5.466207)
  line L1445 (2.432876, -5.466207) -> (2.098167, -5.013579)
  line L1446 (2.098167, -5.013579) -> (1.903667, -4.272534)
  line L1447 (1.903667, -4.272534) -> (2.051495, -3.487293)
  line L1448 (2.051495, -3.487293) -> (2.427732, -2.934272)
  line L1449 (2.427732, -2.934272) -> (2.596325, -2.805875)
  line L1450 (2.596325, -2.805875) -> (3.382709, -2.657285)
  line L1451 (3.382709, -2.657285) -> (3.809429, -2.90322)
  line L1452 (3.809429, -2.90322) -> (3.837432, -2.702624)
  line L1453 (3.837432, -2.702624) -> (3.792093, -2.084642)
  line L1454 (3.792093, -2.084642) -> (3.49758, -1.562672)
  line L1455 (3.49758, -1.562672) -> (2.978658, -1.279589)
  line L1456 (2.978658, -1.279589) -> (2.462022, -1.185291)
  line L1457 (2.462022, -1.185291) -> (2.289239, -1.179195)
  line L1458 (2.289239, -1.179195) -> (2.020633, -1.011746)
  line L1459 (2.020633, -1.011746) -> (1.109853, -0.676085)
  line L1460 (1.109853, -0.676085) -> (-0.02267, -0.608838)
  line L1461 (-0.02267, -0.608838) -> (-1.061466, -0.920687)
  line L1462 (-1.061466, -0.920687) -> (-1.959483, -1.555433)
  line L1463 (-1.959483, -1.555433) -> (-2.670619, -2.454593)
  line L1464 (-2.670619, -2.454593) -> (-3.148012, -3.562541)
  line L1465 (-3.148012, -3.562541) -> (-3.344608, -4.820412)
  line L1466 (-3.344608, -4.820412) -> (-3.287649, -5.843588)
  line L1467 (-3.287649, -5.843588) -> (-3.213354, -6.1722)
  line L1468 (-3.213354, -6.1722) -> (-3.182112, -6.310884)
  line L1469 (-3.182112, -6.310884) -> (-3.203829, -6.785229)
  line L1470 (-3.203829, -6.785229) -> (-3.458146, -7.027926)
  line L1471 (-3.458146, -7.027926) -> (-3.54311, -7.050596)
  line L1472 (-3.54311, -7.050596) -> (-3.686746, -7.087934)
  line L1473 (-3.686746, -7.087934) -> (-4.161854, -7.030974)
  line L1474 (-4.161854, -7.030974) -> (-4.604194, -6.670358)
  line L1475 (-4.604194, -6.670358) -> (-4.868799, -6.078284)
  line L1476 (-4.868799, -6.078284) -> (-4.95662, -5.54374)
  line L1477 (-4.95662, -5.54374) -> (-4.95662, -5.366004)
  line L1478 (-4.95662, -5.366004) -> (-4.946332, 11.406949)
  line L1479 (-4.946332, 11.406949) -> (-5.183124, 11.415522)
  line L1480 (-5.183124, 11.415522) -> (-6.291072, 11.397805)
  line L1481 (-6.291072, 11.397805) -> (-7.302055, 11.298555)
  line L1482 (-7.302055, 11.298555) -> (-7.490079, 11.265408)
  line L1483 (-7.490079, 11.265408) -> (-7.564374, 4.981575)
  line L1484 (-7.564374, 4.981575) -> (-9.394889, 10.648378)
  line L1485 (-9.394889, 10.648378) -> (-9.64692, 10.516171)
  line L1486 (-9.64692, 10.516171) -> (-10.711434, 9.628441)
  line L1487 (-10.711434, 9.628441) -> (-11.522964, 8.418957)
  line L1488 (-11.522964, 8.418957) -> (-11.648884, 8.12673)
  line L1489 (-11.648884, 8.12673) -> (-10.004488, 1.311592)
  line L1490 (-10.004488, 1.311592) -> (-12.356782, 5.399151)
  line L1491 (-12.356782, 5.399151) -> (-12.395073, 5.176837)
  line L1492 (-12.395073, 5.176837) -> (-12.528423, 3.988308)
  line L1493 (-12.528423, 3.988308) -> (-12.584239, 2.814447)
  line L1494 (-12.584239, 2.814447) -> (-12.584239, 2.422588)
  line L1495 (-12.584239, 2.422588) -> (-17.341596, 2.422588)
  line L1496 (-17.341596, 2.422588) -> (-17.341596, 16.11268)
  line L1497 (-17.341596, 16.11268) -> (17.172051, 16.11268)
extrude "Extrusion2" cut sketch "Sketch3 outline for Extrusion2" against normal blind 6.35 keep common part
body "Solid1"
